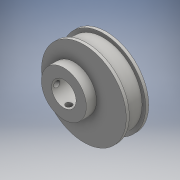
# Autodesk Inventor part: Assieme eccentrico
Saved by Autodesk Inventor 2016 (Build 200138000, 138)
## iProperties
Created: 2016-12-04
Part Number: Assieme eccentrico
Material: Generic
Document SubType Name: Modeling
Designer: Muhammad
Density: 1 g/cm^3
Appearance: Default
Author: Muhammad
Autodesk Inventor part; units mm, degrees
ref_plane "YZ Plane" through (0, 0, 0) normal (1, 0, 0) x (0, 1, 0)
ref_plane "XZ Plane" through (0, 0, 0) normal (0, 1, 0) x (-1, 0, 0)
ref_plane "XY Plane" through (0, 0, 0) normal (0, 0, 1) x (1, 0, 0)
sketch "Sketch1" plane through (0, 0, 0) normal (0, 1, 0) x (-1, 0, 0)
  circle A0 centre (0, 0) radius 20.75
  dimension "d0" = 41.5
  constraints: 1 centre point, 1 coincident
  measures "d0" diameter of A0
extrude "Extrusion1" add sketch "Sketch1" along normal blind 1.5
sketch "Sketch2" plane through (0, 1.5, 0) normal (0, 1, 0) x (1, 0, 0)
  circle A0 centre (0, 0) radius 19
  dimension "d3" = 38
  constraints: 1 centre point, 1 coincident
  measures "d3" diameter of A0
extrude "Extrusion2" add sketch "Sketch2" along normal blind 8
sketch "Sketch3" plane through (0, 9.5, 0) normal (0, 1, 0) x (1, 0, 0)
  circle A0 centre (0, 0) radius 20.75
  constraints: 1 centre point, 1 coincident
extrude "Extrusion3" add sketch "Sketch3" along normal blind 1.5
sketch "Sketch4" plane through (0, 11, 0) normal (0, 1, 0) x (1, 0, 0)
  line L0 (0, 0) -> (-15, 0)
  circle A0 centre (-15, 0) radius 1.6
  line L1 (0, 0) -> (15, 0)
  circle A1 centre (15, 0) radius 1.6
  dimension "d8" = 15
  dimension "d9" = 3.2
  dimension "d10" = 15
  constraints: 4 end point, 2 centre point, 2 coincident, 2 horizontal
  measures "d8" distance of L0.start L0.end
  measures "d9" diameter of A0
  measures "d10" distance of L0.start L1.end
hole "Hole1" at (-15, 11, 0) at (15, 11, 0) direction (0, -1, 0) diameter 3 depth 8 tip angle 118 counterbore diameter 3.2 counterbore depth 6
sketch "Sketch5" plane through (0, 0, 0) normal (0, -1, 0) x (1, 0, 0)
  line L0 (0, 0) -> (-4.8, 0)
  circle A0 centre (-4.8, 0) radius 11
  dimension "d18" = 4.8
  dimension "d19" = 22
  constraints: 2 end point, 1 centre point, 1 coincident, 1 horizontal
  measures "d18" distance of L0.start L0.end
  measures "d19" diameter of A0
extrude "Extrusion4" add sketch "Sketch5" along normal blind 5
sketch "Sketch6" plane through (-4.8, -5, 0) normal (0, -1, 0) x (1, 0, 0)
  circle A0 centre (0, 0) radius 6
  point P0 (4.8, 0)
  dimension "d22" = 12
  constraints: 1 centre point
  measures "d22" diameter of A0
extrude "Extrusion5" cut sketch "Sketch6" against normal through all
sketch "Sketch8" plane through (0, 0, 0) normal (1, 0, 0) x (0, 1, 0)
  line L0 (-5, -6) -> (-5, 6) projected
  line L1 (-5, 0) -> (-2.5, 0)
  circle A0 centre (-2.5, 0) radius 1.5
  point P0 (0, 0)
  dimension "d25" = 2.5
  dimension "d26" = 3
  constraints: 2 end point, 1 centre point, 1 coincident, 1 horizontal, 1 midpoint
  measures "d25" distance of L1.start L1.end
  measures "d26" diameter of A0
extrude "Extrusion6" cut sketch "Sketch8" against normal through all
sketch "Sketch9" plane through (0, 0, 0) normal (0, 0, 1) x (1, 0, 0)
  line L0 (6.2, 0) -> (6.2, -5) projected
  line L1 (6.2, -2.5) -> (-4.8, -2.5)
  circle A0 centre (-4.8, -2.5) radius 1.5
  point P0 (0, 0)
  dimension "d29" = 11
  dimension "d30" = 3
  constraints: 2 end point, 1 centre point, 1 coincident, 1 horizontal, 1 midpoint
  measures "d29" distance of L1.start L1.end
  measures "d30" diameter of A0
extrude "Extrusion7" cut sketch "Sketch9" against normal through all
body "Solid1"
